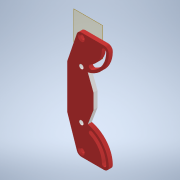
# Autodesk Inventor part: laser_krepl_2
Saved by Autodesk Inventor 2022 (Build 260153000, 153)
## iProperties
Created: 2023-01-26
Part Number: laser_krepl_2
Material: Типовые
Document SubType Name: Modeling
Designer: akapu
Density: 1 g/cm^3
Appearance: По умолчанию
Author: akapu
Autodesk Inventor part; units mm, degrees
ref_plane "YZ Plane" through (0, 0, 0) normal (1, 0, 0) x (0, 1, 0)
ref_plane "XZ Plane" through (0, 0, 0) normal (0, 1, 0) x (-1, 0, 0)
ref_plane "XY Plane" through (0, 0, 0) normal (0, 0, 1) x (1, 0, 0)
ref_plane "РабПлоскость1" through (143.6513, 33.4213, 0) normal (0, 0, 1) x (1, 0, 0)
sketch "Эскиз1" plane through (143.6513, 33.4213, 0) normal (0, 0, 1) x (1, 0, 0)
  line L0 (-148.6513, -34.4651) -> (-94.5662, -34.4651) projected
  circle A0 centre (-2.1213, -2.1213) radius 3.5
  line L1 (1.3787, -2.1213) -> (1.3787, -75.1213)
  line L2 (-5.6213, -75.1213) -> (-5.6213, -2.1213)
  line L3 (-5.6213, -2.7558) -> (-5.6213, -2.1213) projected
  arc A1 (-5.6213, -2.1213) -> (-4.5962, -4.5962) centre (-2.1213, -2.1213) ccw projected
  line L4 (-4.5962, -4.5962) -> (7.3221, -16.5145) projected
  arc A2 (7.3221, -16.5145) -> (12.5466, -11.8741) centre (9.797, -14.0396) ccw projected
  line L5 (12.5466, -11.8741) -> (9.797, -8.3828) projected
  line L6 (9.797, -8.3828) -> (-8.3828, 9.797) projected
  line L7 (-8.3828, 9.797) -> (-9.797, 8.3828) projected
  line L8 (-9.797, 8.3828) -> (-5.6213, -2.7558) projected
  circle A3 centre (-2.1213, -2.1213) radius 1.6 projected
  circle A4 centre (9.797, -14.0396) radius 1.6 projected
  circle A5 centre (-2.1213, -2.1213) radius 16.8551
  line L9 (-2.1213, -2.1213) -> (14.7337, -2.1213)
  line L10 (-2.1213, -2.1213) -> (5.0019, -17.3972)
  line L11 (-2.1213, -2.1213) -> (14.7337, -2.1213) construction
  arc A6 (5.0019, -17.3972) -> (14.7337, -2.1213) centre (-2.1213, -2.1213) ccw construction
  arc A7 (5.6781, -18.8473) -> (16.3337, -2.1213) centre (-2.1213, -2.1213) ccw
  arc A8 (4.3257, -15.9471) -> (13.1337, -2.1213) centre (-2.1213, -2.1213) ccw
  arc A9 (4.3257, -15.9471) -> (5.6781, -18.8473) centre (5.0019, -17.3972) ccw
  arc A10 (16.3337, -2.1213) -> (13.1337, -2.1213) centre (14.7337, -2.1213) ccw
  circle A11 centre (14.7337, -2.1213) radius 3.5
  circle A12 centre (-2.1213, -2.1213) radius 20.3551
  circle A13 centre (-2.1213, -75.1213) radius 20.3551
  line L12 (14.7337, 1.3787) -> (-2.1213, 1.3787)
  line L13 (-5.6213, -38.6213) -> (-12.6213, -38.6213)
  line L14 (2.664, -21.9059) -> (6.8787, -32.8062)
  line L15 (6.8787, -32.8062) -> (6.8787, -44.0201)
  line L16 (6.8787, -44.0201) -> (2.6355, -55.3299)
  line L17 (-12.6213, -38.6213) -> (-12.6213, -54.8947)
  line L18 (-12.6213, -54.8947) -> (-5.6213, -59.1452)
  line L19 (-12.6213, -38.6213) -> (-12.6213, -22.3479)
  line L20 (-12.6213, -22.3479) -> (-5.6213, -18.072)
  circle A14 centre (9.7969, -63.2026) radius 1.6 projected
  circle A15 centre (-2.1214, -75.1214) radius 16.8553
  line L21 (-2.1214, -75.1214) -> (5.002, -59.8453)
  line L22 (-2.1214, -75.1214) -> (14.7339, -75.1214) construction
  line L23 (-2.1214, -75.1214) -> (14.7339, -75.1214)
  arc A16 (14.7339, -75.1214) -> (5.002, -59.8453) centre (-2.1214, -75.1214) ccw construction
  arc A17 (16.3339, -75.1214) -> (5.6782, -58.3952) centre (-2.1214, -75.1214) ccw
  arc A18 (13.1339, -75.1214) -> (4.3258, -61.2954) centre (-2.1214, -75.1214) ccw
  arc A19 (13.1339, -75.1214) -> (16.3339, -75.1214) centre (14.7339, -75.1214) ccw
  arc A20 (5.6782, -58.3952) -> (4.3258, -61.2954) centre (5.002, -59.8453) ccw
  circle A21 centre (14.7339, -75.1214) radius 3.5
  line L24 (14.7339, -78.6214) -> (-2.1213, -78.6213)
  line L25 (-8.3825, -87.0398) -> (9.7969, -68.8596) projected
  line L26 (9.7969, -68.8596) -> (12.5465, -65.3681) projected
  arc A22 (12.5465, -65.3681) -> (7.3219, -60.7278) centre (9.7969, -63.2026) ccw projected
  line L27 (7.3219, -60.7278) -> (-4.5962, -72.6465) projected
  arc A23 (-4.5962, -72.6465) -> (-5.3987, -73.8929) centre (-2.1214, -75.1214) ccw projected
  line L28 (-5.3987, -73.8929) -> (-9.7968, -85.6256) projected
  line L29 (-9.7968, -85.6256) -> (-8.3825, -87.0398) projected
  circle A24 centre (9.7969, -63.2026) radius 1.6 projected
  circle A25 centre (-2.1214, -75.1214) radius 1.6 projected
  circle A26 centre (-2.1214, -75.1214) radius 3.4999
  line L30 (-12.6213, -22.3479) -> (-5.4385, -1.0049)
  line L31 (-12.6213, -54.8947) -> (-5.4385, -76.2377)
  ellipse E0 centre (-92.9013, -13.3149) end of major axis (-92.9013, -38.7397) minor radius 3 (-94.5662, -34.4651) -> (-93.1905, -38.6213) ccw projected
  line L32 (-148.6513, -42.7775) -> (-148.6513, -34.4651) projected
  line L33 (-94.5662, -42.7775) -> (-148.6513, -42.7775) projected
  ellipse E1 centre (-92.9013, -63.9277) end of major axis (-92.9013, -38.5029) minor radius 3 (-93.1905, -38.6213) -> (-94.5662, -42.7775) ccw projected
  circle A27 centre (-2.1213, -56.6213) radius 1.6
  circle A28 centre (-2.1213, -20.6213) radius 1.6
  point P0 (-143.6513, -33.4213)
  point P1 (1.3787, -2.1213)
  point P2 (14.3665, -78.6214)
  point P3 (14.3706, -78.6025)
  point P4 (18.2337, -75.1631)
  point P5 (1.3787, -55.0694)
  point P6 (1.3787, -22.1732)
  point P7 (18.2337, -2.1213)
  point P8 (14.3703, 1.3598)
  point P9 (14.3663, 1.3787)
  point P10 (1.3787, -67.6155)
  point P11 (4.3258, -61.2954)
  point P12 (12.8465, -72.1739)
  point P13 (1.3787, -18.609)
  point P14 (1.3787, -58.6335)
  point P15 (-2.1213, -78.6213)
  point P16 (4.3258, -61.2954)
  point P17 (-5.8355, -75.0581)
  point P18 (-5.6213, -74.4868)
  point P19 (-5.8355, -2.1845)
  point P20 (-5.6213, -22.1732)
  point P21 (-5.6213, -55.0694)
  point P22 (-10.1295, -56.4078)
  point P23 (-5.6213, -58.6334)
  point P24 (-2.1213, -78.6213)
  dimension "d6" = 7
  dimension "d10" = 7
  dimension "d3" = 65
  dimension "d7" = 7
  dimension "d9" = 65
  constraints: 40 end point, 31 point on circle, 15 centre point, 13 tangent, 5 coincident, 5 horizontal, 3 point on line, 2 equal length, 2 parallel, 1 collinear, 1 midpoint, 22 other
  measures "d3" angle of L10 L11
  measures "d7" distance of L13.start L13.end
  measures "d9" angle of L22 L21
extrude "Выдавливание1" add sketch "Эскиз1" along normal blind 3 contours L9 A3 L10 A0 | L1 L10 A0 | L9 L6 L5 A8 L4 L10 L1 | A0 L10 A3 L9 | A0 L12 L6 L9 | L10 L1 L4 A0 | L10 L4 L1 | L9 A11 A8 L5 L6 | L6 L12 A5 A11 L9 | A0 L2 L8 L30 | L4 L1 A5 L2 A0 | L4 L10 A9 A5 L1 | L4 A8 L10 | A11 A5 A10 L9 | L9 A8 A11 | L8 L2 L20 A5 L30 | L12 A11 A5 | A5 A9 A7 A2 A12 L1 | L1 A12 L2 A5 | A11 A7 A10 A5 | A5 L20 A12 L30 | A12 L14 L15 L16 A13 L1 | L1 A13 L2 A12 | A5 L20 L2 | L2 A12 L20 A5 | A12 L20 L30 | A12 A2 A7 A11 | A13 A22 A17 A20 A15 L1 | L1 A15 L2 A13 | L2 L13 L19 L20 A12 | A2 A7 | A15 A20 L21 L27 L1 | L1 L27 A23 L28 L2 A15 | A13 L18 L17 L13 L2 | L2 A15 L18 A13 | L27 L21 L1 | L1 L21 A26 L27 | L2 L18 A15 | A13 A21 A17 A22 | A22 A17 | L18 A15 L31 A13 | A13 L31 L18 | L21 L27 A18 L26 L25 L23 L1 | L1 A26 L21 | L21 A18 L27 | A26 L21 A25 L23 A23 | L2 L28 L31 A15 L18 | A21 A15 A19 A17 | L23 L25 L24 A26 | L23 A25 L21 A26 | A26 L2 L28 | L2 A26 L31 L28 | L24 A15 A21 | L25 L26 A18 A21 L23 | L23 A21 A15 L24 L25 | A21 L23 A19 A15 | A21 A18 L23 picked at (16.9237, -2.7577) picked at (16.9239, -74.485)
chamfer "Фаска1" distance 0.9 angle 45 2 edges at (139.93, 31.3, 3) (139.9299, -41.7001, 3)
